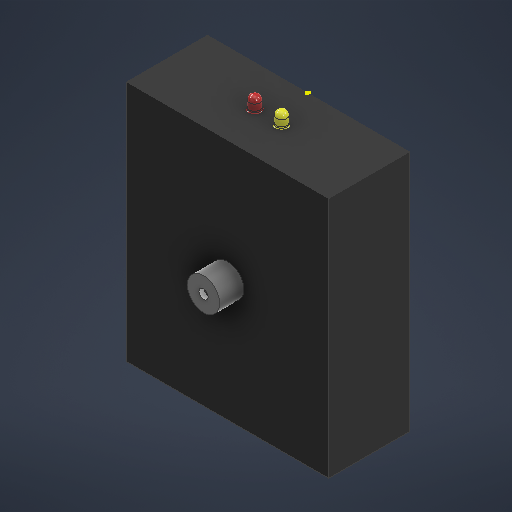
# Autodesk Inventor part: Utuh
Saved by Autodesk Inventor 2027 (Build 310192000, 192)
## iProperties
Created: 2026-06-02
Part Number: Utuh
Material: Generic
Document SubType Name: Sheet Metal
Designer: acer
Density: 1 g/cm^3
Sheet Metal Rule: Default_mm
Appearance: Default
Author: acer
Autodesk Inventor part; units mm, degrees
ref_plane "YZ Plane" through (0, 0, 0) normal (1, 0, 0) x (0, 1, 0)
ref_plane "XZ Plane" through (0, 0, 0) normal (0, 1, 0) x (-1, 0, 0)
ref_plane "XY Plane" through (0, 0, 0) normal (0, 0, 1) x (1, 0, 0)
sketch "Sketch1" plane through (0, 0, 0) normal (0, 0, 1) x (1, 0, 0)
  line L0 (-37.5, 45) -> (37.5, 45)
  line L1 (37.5, 45) -> (37.5, -45)
  line L2 (37.5, -45) -> (-37.5, -45)
  line L3 (-37.5, -45) -> (-37.5, 45)
  point P0 (0, 0)
  point P1 (0, -45)
  point P2 (0, 45)
  point P3 (-37.5, 0)
  dimension "d0" = 90
  dimension "d1" = 75
  dimension "d2" = 37.5
  dimension "d3" = 45
  constraints: 8 end point, 3 midpoint, 2 parallel, 1 horizontal, 1 perpendicular
  measures "d0" distance of point (0, -45) point (0, 45)
  measures "d1" distance between parallel lines of L1 L3
  measures "d2" distance of point (0, 0) point (-37.5, 0)
  measures "d3" distance of point (0, -45) point (0, 0)
extrude "Extrusion1" add sketch "Sketch1" along normal blind 30
shell "Shell1" thickness 2 removed faces 0
sketch "Sketch2" plane through (-37.5, 45, 0) normal (0, 1, 0) x (1, 0, 0)
  circle A0 centre (42.5, -15) radius 2
  line L0 (75, 0) -> (0, 0) projected
  circle A1 centre (32.5, -15) radius 2
  line L1 (75, 0) -> (75, -30) projected
  point P0 (37.5, 0)
  point P1 (37.5, 0)
  dimension "d7" = 15
  dimension "d8" = 10
  dimension "d9" = 15
  dimension "d10" = 4
  dimension "d11" = 4
  dimension "d12" = 32.5
  constraints: 2 centre point, 1 midpoint
  measures "d7" distance from line of L0 A0.centre
  measures "d8" distance of A0.centre A1.centre
  measures "d9" vertical distance of point (37.5, 0) A1.centre
  measures "d10" diameter of A0
  measures "d11" diameter of A1
  measures "d12" distance from line of L1 A0.centre
extrude "Extrusion2" add sketch "Sketch2" along normal blind 5
fillet "Fillet1" radius 2 1 edges at (3, 50, 15)
fillet "Fillet2" radius 2 1 edges at (-7, 50, 15)
chamfer "Chamfer1" distance 0.5 angle 45 1 edges at (3, 45, 15)
chamfer "Chamfer2" distance 0.5 angle 45 1 edges at (-7, 45, 15)
fillet "Fillet3" radius 0.5 1 edges at (3, 45.5, 15)
fillet "Fillet4" radius 0.5 1 edges at (-7, 45.5, 15)
sketch "Sketch3" plane through (0, 0, 30) normal (0, 0, 1) x (1, 0, 0)
  circle A0 centre (0, 0) radius 6
  dimension "d25" = 12
  constraints: 1 centre point, 1 coincident
  measures "d25" diameter of A0
extrude "Extrusion3" add sketch "Sketch3" along normal blind 9
sketch "Sketch4" plane through (0, 0, 39) normal (0, 0, 1) x (1, 0, 0)
  circle A0 centre (0, 0) radius 1.75
  dimension "d28" = 3.5
  constraints: 1 centre point, 1 coincident
  measures "d28" diameter of A0
extrude "Extrusion4" cut sketch "Sketch4" against normal blind 2
sketch "Sketch5" plane through (-37.5, 45, 0) normal (0, 1, 0) x (1, 0, 0)
  point P0 (37.5, 0)
sketch "Sketch6" plane through (-37.5, -45, 0) normal (-1, 0, 0) x (0, 0, 1)
  line L0 (25, 57.1263) -> (5, 57.1263)
  line L1 (5, 57.1263) -> (5, 24.9712)
  line L2 (5, 24.9712) -> (25, 24.9712)
  line L3 (25, 24.9712) -> (25, 57.1263)
  line L4 (30, 90) -> (30, 0) projected
  line L5 (0, 90) -> (0, 0) projected
  point P0 (0, 45)
  point P1 (25, 41.0487)
  dimension "d31" = 5
  dimension "d32" = 5
  constraints: 8 end point, 2 parallel, 1 horizontal, 1 midpoint, 1 perpendicular
  measures "d31" distance from line of point (25, 41.049) L4
  measures "d32" distance between parallel lines of L5 L1
extrude "Extrusion5" cut sketch "Sketch6" against normal blind 2
sketch "Sketch7" plane through (-37.5, -45, 0) normal (-1, 0, 0) x (0, 0, 1)
  point P0 (0, 45)
equation "\"BendRadius\" = Thickness"
equation "\"BendReliefWidth\" = Thickness"
equation "\"BendReliefDepth\" = 0.5 * Thickness"
equation "\"CornerReliefSize\" = 4 * Thickness"
equation "\"MinimumRemnant\" = 2 * Thickness"
equation "\"TransitionRadius\" = BendRadius"
equation "\"JacobiRadiusSize\" = BendRadius"
equation "\"GapSize\" = Thickness"
equation "\"Thickness\" = 0.5"
body "Solid1"
